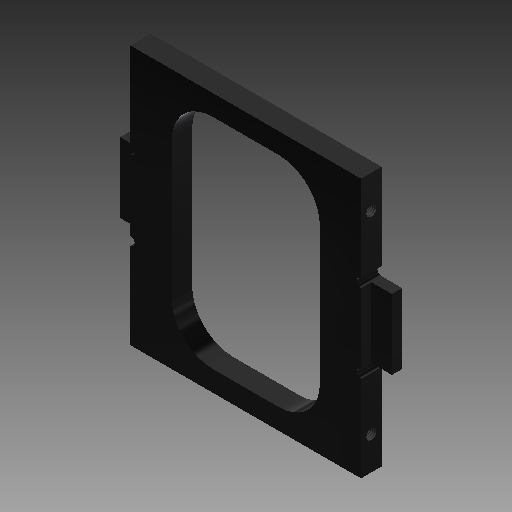
# Autodesk Inventor part: コックピット_2_サブフレーム_4
Saved by Autodesk Inventor 2018 (Build 220112000, 112)
## iProperties
Created: 2016-05-24
Part Number: コックピット_2_サブフレーム_4
Material: アセタール樹脂、黒
Document SubType Name: Modeling
Designer: hiroaki
Density: 1.425 g/cm^3
Appearance: 滑らか - 黒
Mass: 12.6427 g
Surface Area: 58.8321 cm^2
Volume: 8.87208 cm^3
Author: hiroaki
Autodesk Inventor part; units mm, degrees
ref_plane "YZ Plane" through (0, 0, 0) normal (1, 0, 0) x (0, 1, 0)
ref_plane "XZ Plane" through (0, 0, 0) normal (0, 1, 0) x (-1, 0, 0)
ref_plane "XY Plane" through (0, 0, 0) normal (0, 0, 1) x (1, 0, 0)
sketch "スケッチ1" plane through (0, 0, 0) normal (0, 0, 1) x (1, 0, 0)
  line L0 (-28, -31.5) -> (28, -31.5) construction
  line L1 (28, -31.5) -> (28, 31.5) construction
  line L2 (28, 31.5) -> (-28, 31.5) construction
  line L3 (-28, 31.5) -> (-28, -31.5) construction
  line L4 (-28, -31.5) -> (28, 31.5) construction
  line L5 (28, -31.5) -> (-28, 31.5) construction
  line L6 (-28, 10.6) -> (-28, 31.5)
  line L7 (-28, 31.5) -> (28, 31.5)
  line L8 (28, 31.5) -> (28, 10.6)
  line L9 (-28, -10.6) -> (-28, -31.5)
  line L10 (-28, -31.5) -> (28, -31.5)
  line L11 (28, -31.5) -> (28, -10.6)
  line L12 (-28, 8.5) -> (-33, 8.5)
  line L13 (-33, 8.5) -> (-33, -8.5)
  line L14 (-33, -8.5) -> (-28, -8.5)
  line L15 (28, 8.5) -> (33, 8.5)
  line L16 (33, 8.5) -> (33, -8.5)
  line L17 (33, -8.5) -> (28, -8.5)
  line L18 (0, 0) -> (0, 31.5) construction
  line L19 (0, 0) -> (28, 0) construction
  arc A0 (-28, 8.5) -> (-28, 10.6) centre (-28, 9.55) ccw
  arc A1 (-28, -10.6) -> (-28, -8.5) centre (-28, -9.55) ccw
  arc A2 (28, 10.6) -> (28, 8.5) centre (28, 9.55) ccw
  arc A3 (28, -8.5) -> (28, -10.6) centre (28, -9.55) ccw
  dimension "d45" = 63
  dimension "d73" = 56
  dimension "d74" = 1.05
  dimension "d75" = 5
  dimension "d76" = 23
  constraints: 40 end point, 8 perpendicular, 8 point on circle, 4 centre point, 4 midpoint, 4 symmetric about line, 4 tangent, 3 collinear, 3 horizontal, 3 vertical, 3 vertical alignment, 2 parallel, 1 equal radius, 2 other
  measures "d45" distance of L2.end L0.start
  measures "d73" distance of L1.end L2.end
  measures "d74" radius of A0
  measures "d75" distance between parallel lines of L13 L3
  measures "d76" distance between parallel lines of L7 L12
extrude "押し出し1" add sketch "スケッチ1" along normal blind 5
sketch "スケッチ2" plane through (0, 0, 5) normal (0, 0, 1) x (1, 0, 0)
  line L0 (-28, 31.5) -> (-28, 10.6) projected
  line L1 (28, 10.6) -> (28, 31.5) projected
  line L2 (-50.9845, 57.5344) -> (-28, 57.5344)
  line L3 (-28, 57.5344) -> (-28, -57.37)
  line L4 (-28, -57.37) -> (-50.9845, -57.37)
  line L5 (-50.9845, -57.37) -> (-50.9845, 57.5344)
  line L6 (28, 64.7229) -> (65.0267, 64.7229)
  line L7 (65.0267, 64.7229) -> (65.0267, -57.37)
  line L8 (65.0267, -57.37) -> (28, -57.37)
  line L9 (28, -57.37) -> (28, 64.7229)
  point P0 (0, 0)
  constraints: 16 end point, 4 parallel, 2 collinear, 2 horizontal, 2 perpendicular, 1 point on line
extrude "押し出し2" cut sketch "スケッチ2" against normal blind 2.5
sketch "スケッチ3" plane through (28, -31.5, 0) normal (1, 0, 0) x (0, 0, -1)
  line L0 (0, 0) -> (-5, 0) projected
  line L1 (0, 63) -> (-5, 63) projected
  point P0 (0, 31.5)
  point P1 (-2.5, 8)
  point P2 (-2.5, 55)
  point P3 (-2.5, 0)
  dimension "d81" = 8
  dimension "d82" = 8
  constraints: 2 vertical alignment, 1 midpoint
  measures "d81" distance from line of L0 point (-2.5, 8)
  measures "d82" distance from line of L1 point (-2.5, 55)
hole "穴1" at (28, -23.5, 2.5) at (28, 23.5, 2.5) direction (-1, 0, 0) diameter 2.459 depth 2.5 thread size "M3x0.5" class "6H" standard "ISO Metric profile"
mirror "ミラー1" about plane through (0, 0, 0) normal (1, 0, 0) of "穴1"
sketch "スケッチ4" plane through (0, 0, 5) normal (0, 0, 1) x (1, 0, 0)
  line L0 (-28, -31.5) -> (28, -31.5) projected
  line L1 (28, -31.5) -> (28, -10.6) projected
  line L2 (18, 26.5) -> (-18, 26.5)
  line L3 (-18, 26.5) -> (-18, -26.5)
  line L4 (-18, -26.5) -> (18, -26.5)
  line L5 (18, -26.5) -> (18, 26.5)
  line L6 (18, 26.5) -> (-18, -26.5) construction
  line L7 (-18, 26.5) -> (18, -26.5) construction
  point P0 (0, 0)
  dimension "d90" = 10
  dimension "d91" = 5
  constraints: 12 end point, 2 midpoint, 2 parallel, 1 horizontal, 1 perpendicular
  measures "d90" distance between parallel lines of L1 L5
  measures "d91" distance between parallel lines of L0 L4
extrude "押し出し3" cut sketch "スケッチ4" against normal blind 10
fillet "フィレット1" radius 10 4 edges at (18, -26.5, 2.5) (-18, -26.5, 2.5) (-18, 26.5, 2.5) (18, 26.5, 2.5)
equation "\"d45\" = d1"
equation "\"d76\" = d20 + d23"
equation "\"d81\" = d20"
equation "\"d82\" = d81"
equation "\"d1\" = 63"
equation "\"d20\" = 8"
equation "\"d23\" = 15"
